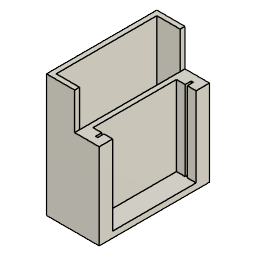
Drybox_Device_Holder_v56 (Autodesk Fusion 360 design; units mm, degrees)
Autodesk Fusion 360 part; units mm, degrees
sketch "Sketch1" plane through (0, 0, 0) normal (0, 0, 1) x (1, 0, 0)
  line L0 (0, 0) -> (20, 0)
  line L1 (20, 90) -> (0, 90)
  line L2 (0, 90) -> (0, 0)
  line L3 (4, 79) -> (11.125, 79)
  line L4 (11.125, 79) -> (11.125, 84)
  line L5 (4, 11) -> (4, 79)
  line L6 (0, 75) -> (0, 25)
  line L7 (20, 90) -> (0, 0) construction
  line L8 (0, 90) -> (20, 0) construction
  line L9 (0, 90) -> (-23, 90)
  line L10 (-23, 90) -> (-23, 0)
  line L11 (-23, 0) -> (0, 0)
  line L12 (0, 0) -> (0, 90)
  line L13 (0, 90) -> (-23, 0) construction
  line L14 (-23, 90) -> (0, 0) construction
  line L15 (10, 45) -> (-11.5, 45) construction
  line L16 (0, 86) -> (-19, 86)
  line L17 (-19, 86) -> (-19, 4)
  line L18 (-19, 4) -> (0, 4)
  line L19 (12, 90) -> (12, 0) construction
  line L20 (11.125, 84) -> (12, 84)
  line L21 (20, 79) -> (12.875, 79)
  line L22 (12.875, 79) -> (12.875, 84)
  line L23 (12.875, 84) -> (12, 84)
  line L24 (20, 90) -> (20, 0)
  line L25 (20, 11) -> (12.875, 11)
  line L26 (4, 11) -> (11.125, 11)
  line L27 (11.125, 11) -> (11.125, 6)
  line L28 (11.125, 6) -> (12, 6)
  line L29 (12.875, 6) -> (12, 6)
  line L30 (12.875, 11) -> (12.875, 6)
  point P0 (-11.5, 45)
  dimension "d37" = 90
  dimension "d38" = 23
  dimension "d39" = -4
  dimension "d51" = 12
  dimension "d57" = 1.75
  dimension "d63" = 5
  dimension "d65" = 78
  dimension "d66" = 6
  dimension "d67" = 20
  dimension "d72" = 8
  constraint horizontal L0
  constraint horizontal L1
  constraint vertical L2
  constraint coincident L0.start L2.end
  constraint horizontal L3
  constraint perpendicular L3 L4
  constraint perpendicular L3 L5
  constraint vertical L6
  constraint coincident L2 L6.end
  constraint horizontal L9
  constraint perpendicular L9 L10
  constraint parallel L9 L11
  constraint parallel L10 L12
  constraint coincident L13 P0
  constraint coincident L14 P0
  constraint coincident L2 L1.end
  constraint midpoint L7 L15.start
  constraint coincident P0 L15.end
  constraint horizontal L15
  constraint coincident L1 L19.start
  constraint coincident L0 L19.end
  constraint perpendicular L0 L19
  constraint coincident L19 L20.end
  constraint perpendicular L19 L20
  constraint symmetric L3.start L19 L21.start
  constraint symmetric L3.end L19 L21.end
  constraint symmetric L4.end L19 L22.end
  constraint symmetric L19 L20.end L23.end
  constraint symmetric L3.start L15 L5.start
  constraint symmetric L3.end L15 L26.end
  constraint symmetric L4.end L15 L27.end
  constraint symmetric L15 L20.end L28.end
  constraint symmetric L15 L21.start L25.start
  constraint symmetric L15 L21.end L25.end
  constraint symmetric L15 L22.end L29.start
  measures "d37" distance of L9.end L10.end
  measures "d38" distance of L10.end L0.start
  measures "d51" distance of L2 L19
  measures "d57" distance of L4 L22
  measures "d63" distance of L21.end L22.end
  measures "d65" distance of L20 L28
  measures "d66" distance of L1 L20
  measures "d67" distance of L2 L24
  measures "d72" distance of L5 L19
extrude "Extrude7" add sketch "Sketch1" along normal blind 5 contours L2 L6 L12 L16 L17 L18 | L3 L4 L5 L20 L21 L22 L23 L24 L25 L26 L27 L28 L29 L30 makes body 1 at (6.375, 33.6667, 0) makes body 2 at (-6.3333, 58.6667, 0)
extrude "Extrude9" add sketch "Sketch1" along normal blind 70 contours L0 L1 L2 L3 L4 L5 L6 L12 L20 L21 L22 L23 L24 L25 L26 L27 L28 L29 L30 bodies 1 2
extrude "Extrude10" add sketch "Sketch1" along normal blind 100 contours L2 L9 L10 L11 L12 L16 L17 L18 bodies 1
